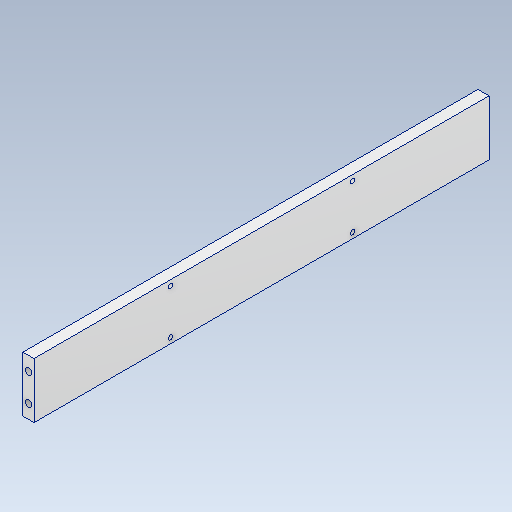
# Autodesk Inventor part: Travesaño Estructural
Saved by Autodesk Inventor 2020 (Build 240168000, 168)
## iProperties
Created: 2020-05-17
Part Number: Travesaño Estructural
Material: Aluminum 6061
Document SubType Name: Modeling
Designer: Dante
Density: 2.7 g/cm^3
Appearance: Aluminum - Flat
Author: Dante
Autodesk Inventor part; units mm, degrees
ref_plane "YZ Plane" through (0, 0, 0) normal (1, 0, 0) x (0, 1, 0)
ref_plane "XZ Plane" through (0, 0, 0) normal (0, 1, 0) x (-1, 0, 0)
ref_plane "XY Plane" through (0, 0, 0) normal (0, 0, 1) x (1, 0, 0)
sketch "Sketch1" plane through (0, 0, 0) normal (0, 0, 1) x (1, 0, 0)
  line L0 (0, 0) -> (0, -50)
  line L1 (0, -50) -> (10, -50)
  line L2 (10, -50) -> (10, 0)
  line L3 (10, 0) -> (0, 0)
  dimension "d1" = 50
  dimension "d2" = 10
  constraints: 8 end point, 3 perpendicular, 1 vertical
  measures "d1" distance of L0.start L0.end
  measures "d2" distance of L0.end L1.end
extrude "Extrusion1" add sketch "Sketch1" along normal blind 410
sketch "Sketch2" plane through (0, 0, 0) normal (0, 0, -1) x (-1, 0, 0)
  circle A0 centre (-5, -12.5) radius 3
  circle A1 centre (-5, -37.5) radius 3
  line L0 (-10, -50) -> (-10, 0) projected
  line L1 (-10, 0) -> (0, 0) projected
  line L2 (0, -50) -> (-10, -50) projected
  dimension "d5" = 6
  dimension "d6" = 6
  dimension "d7" = 5
  dimension "d8" = 5
  dimension "d9" = 12.5
  dimension "d10" = 12.5
  constraints: 2 centre point
  measures "d5" diameter of A0
  measures "d6" diameter of A1
  measures "d7" distance from line of L0 A1.centre
  measures "d8" distance from line of L0 A0.centre
  measures "d9" distance from line of L1 A0.centre
  measures "d10" distance from line of L2 A1.centre
sketch "Sketch3" plane through (0, 0, 410) normal (0, 0, 1) x (1, 0, 0)
  circle A0 centre (5, -12.5) radius 3 projected
  circle A1 centre (5, -12.5) radius 3
  circle A2 centre (5, -37.5) radius 3 projected
  circle A3 centre (5, -37.5) radius 3
  point P0 (0, 0)
  constraints: 2 centre point, 2 coincident
hole "Agujero2" at (5, -12.5, 0) at (5, -37.5, 0) direction (0, 0, 1) diameter 6 depth 15 tip angle 118
hole "Agujero3" at (5, -12.5, 410) at (5, -37.5, 410) direction (0, 0, -1) diameter 6 depth 15 tip angle 118
thread "Rosca5" size "M6x1" class "6H" standard "ISO Metric profile" length 10
thread "Rosca6" size "M6x1" class "6H" standard "ISO Metric profile" length 10
thread "Rosca7" size "M6x1" class "6H" standard "ISO Metric profile" length 430
thread "Rosca8" size "M6x1" class "6H" standard "ISO Metric profile" length 430
sketch "Boceto4" plane through (10, -50, 0) normal (1, 0, 0) x (0, 0, -1)
  circle A0 centre (-287, 45) radius 2
  circle A1 centre (-287, 5) radius 2
  circle A2 centre (-123, 5) radius 2
  circle A3 centre (-123, 45) radius 2
  line L0 (-410, 0) -> (-410, 50) projected
  line L1 (0, 0) -> (0, 50) projected
  line L2 (0, 50) -> (-410, 50) projected
  dimension "d52" = 4
  dimension "d53" = 4
  dimension "d54" = 4
  dimension "d55" = 4
  dimension "d56" = 123
  dimension "d57" = 123
  dimension "d60" = 5
  dimension "d63" = 5
  dimension "d74" = 40
  dimension "d75" = 40
  constraints: 4 centre point
  measures "d52" diameter of A0
  measures "d53" diameter of A1
  measures "d54" diameter of A2
  measures "d55" diameter of A3
  measures "d56" distance from line of L0 A0.centre
  measures "d57" distance from line of L1 A3.centre
  measures "d60" distance from line of L2 A0.centre
  measures "d63" distance from line of L2 A3.centre
  measures "d74" distance of A1.centre A0.centre
  measures "d75" distance of A2.centre A3.centre
extrude "Extrusión4" cut sketch "Boceto4" against normal blind 10
equation "\"d63\" = d60"
body "Solid1"
